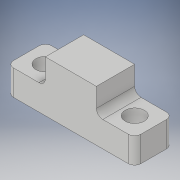
# Autodesk Inventor part: Mirror 3D
Saved by Autodesk Inventor 2017 (Build 210142000, 142)
## iProperties
Created: 2020-02-21
Part Number: Mirror 3D
Material: Generic
Document SubType Name: Modeling
Designer: 10042265
Density: 1 g/cm^3
Appearance: Default
Author: 10042265
Autodesk Inventor part; units mm, degrees
ref_plane "YZ Plane" through (0, 0, 0) normal (1, 0, 0) x (0, 1, 0)
ref_plane "XZ Plane" through (0, 0, 0) normal (0, 1, 0) x (-1, 0, 0)
ref_plane "XY Plane" through (0, 0, 0) normal (0, 0, 1) x (1, 0, 0)
sketch "Sketch1" plane through (0, 0, 0) normal (0, 0, 1) x (1, 0, 0)
  line L0 (0, 0) -> (31.75, 0)
  line L1 (31.75, 0) -> (31.75, 25.4)
  line L2 (31.75, 25.4) -> (19.05, 25.4)
  line L3 (19.05, 25.4) -> (19.05, 12.7)
  line L4 (19.05, 12.7) -> (0, 12.7)
  line L5 (0, 12.7) -> (0, 0)
  dimension "d0" = 31.75
  dimension "d1" = 25.4
  dimension "d2" = 12.7
  dimension "d3" = 12.7
  constraints: 12 end point, 5 perpendicular, 1 horizontal
  measures "d0" distance of L0.start L0.end
  measures "d1" distance of L0.end L1.end
  measures "d2" distance of L1.end L2.end
  measures "d3" distance of L2.end L3.end
extrude "Extrusion1" add sketch "Sketch1" along normal blind 19.05
fillet "Fillet1" radius 3.175 3 edges at (0, 6.35, 19.05) (19.05, 12.7, 9.525) (0, 6.35, 0)
sketch "Sketch2" plane through (3.175, 12.7, 0) normal (0, 1, 0) x (1, 0, 0)
  line L0 (15.875, 0) -> (12.7, 0) projected
  circle A0 centre (6.35, -9.4797) radius 4.7625
  point P0 (-3.175, 0)
  dimension "d7" = 9.525
  constraints: 1 centre point
  measures "d7" diameter of A0
extrude "Extrusion2" cut sketch "Sketch2" against normal blind 12.7
mirror "Mirror1" about plane through (31.75, 0, 0) normal (1, 0, 0) of "Extrusion1", "Extrusion2", "Fillet1"
body "Solid1"
